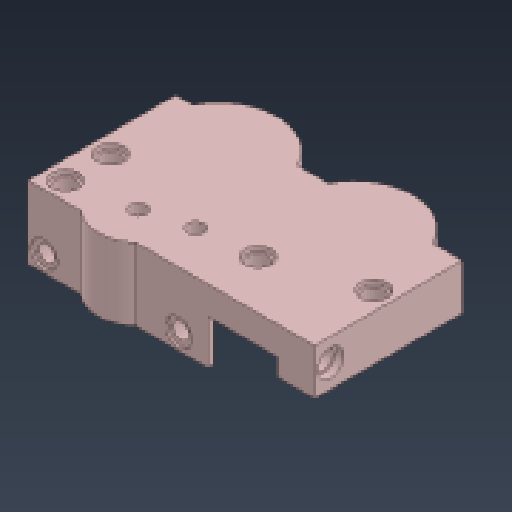
# Autodesk Inventor part: gearbox-holder-right
Saved by Autodesk Inventor 2023 (Build 270158000, 158)
## iProperties
Created: 2025-04-06
Part Number: gearbox-holder-right
Material: ABS Plastic
Document SubType Name: Modeling
Designer: szymo
Density: 1.06 g/cm^3
Appearance: Default(1)
Mass: 8.8839 g
Surface Area: 69.2878 cm^2
Volume: 8.38104 cm^3
Author: szymo
Autodesk Inventor part; units mm, degrees
(part 1 of 3)
ref_plane "YZ Plane" through (0, 0, 0) normal (1, 0, 0) x (0, 1, 0)
ref_plane "XZ Plane" through (0, 0, 0) normal (0, 1, 0) x (-1, 0, 0)
ref_plane "XY Plane" through (0, 0, 0) normal (0, 0, 1) x (1, 0, 0)
ref_plane "Work Plane1" through (-2.05, 16.2, 13.85) normal (0, 1, 0) x (0.7160287, 0, -0.6980708)
sketch "Sketch1" plane through (-2.05, 16.2, 13.85) normal (0, 1, 0) x (0.7160287, 0, -0.6980708)
  line L0 (-0.2487, 19.5853) -> (0.8969, 18.4684) projected
  line L1 (-18.9501, -1.8892) -> (0.8969, 18.4684) projected
  line L2 (-20.0957, -0.7723) -> (-18.9501, -1.8892) projected
  line L3 (-20.0957, -0.7723) -> (-0.2487, 19.5853) projected
  circle A0 centre (0, 8) radius 1.0564 projected
  circle A1 centre (0, -8) radius 1.0564 projected
  circle A2 centre (0, 0) radius 5 projected
  circle A3 centre (0, 0) radius 13.85 projected
  line L4 (0.8969, 18.4684) -> (19.5853, 0.2487)
  line L5 (19.5853, 0.2487) -> (0.2487, -19.5853)
  line L6 (0, 0) -> (9.917, -9.6683) construction
  circle A4 centre (19.834, -19.3366) radius 13.85 projected
  line L7 (19.5853, 0.2487) -> (25.0919, -5.1198)
  circle A5 centre (19.834, -19.3366) radius 14.25
  line L8 (25.0919, -5.1198) -> (24.3938, -5.8358)
  circle A6 centre (-3.741, -7.91) radius 1.25 projected
  arc A7 (-6.4074, -14.111) -> (-5.6342, -13.2068) centre (-9.5026, -10.6812) ccw projected
  arc A8 (-5.6342, -13.2068) -> (-5.2978, -13.3152) centre (-3.741, -7.91) ccw projected
  arc A9 (-5.2978, -13.3152) -> (-5.1983, -14.5008) centre (-0.6827, -13.5245) ccw projected
  arc A10 (-5.1983, -14.5008) -> (-4.7815, -14.5793) centre (-3.741, -7.91) ccw projected
  arc A11 (-4.7815, -14.5793) -> (-4.2574, -13.5112) centre (-8.6325, -12.027) ccw projected
  arc A12 (-4.2574, -13.5112) -> (-3.9047, -13.5326) centre (-3.741, -7.91) ccw projected
  arc A13 (-3.9047, -13.5326) -> (-3.5134, -14.6561) centre (0.6175, -12.5875) ccw projected
  arc A14 (-3.5134, -14.6561) -> (-3.0903, -14.6285) centre (-3.741, -7.91) ccw projected
  arc A15 (-3.0903, -14.6285) -> (-2.8482, -13.4637) centre (-7.4549, -13.1141) ccw projected
  arc A16 (-2.8482, -13.4637) -> (-2.5013, -13.3966) centre (-3.741, -7.91) ccw projected
  arc A17 (-2.5013, -13.3966) -> (-1.8429, -14.3876) centre (1.6439, -11.3566) ccw projected
  arc A18 (-1.8429, -14.3876) -> (-1.4399, -14.2556) centre (-3.741, -7.91) ccw projected
  arc A19 (-1.4399, -14.2556) -> (-1.4951, -13.0672) centre (-6.044, -13.8742) ccw projected
  arc A20 (-1.4951, -13.0672) -> (-1.1757, -12.916) centre (-3.741, -7.91) ccw projected
  arc A21 (-1.1757, -12.916) -> (-0.2916, -13.712) centre (2.3318, -9.9092) ccw projected
  arc A22 (-0.2916, -13.712) -> (0.0659, -13.484) centre (-3.741, -7.91) ccw projected
  arc A23 (0.0659, -13.484) -> (-0.2831, -12.3466) centre (-4.4884, -14.2596) ccw projected
  arc A24 (-0.2831, -12.3466) -> (-0.0114, -12.1207) centre (-3.741, -7.91) ccw projected
  arc A25 (-0.0114, -12.1207) -> (1.043, -12.6719) centre (2.6382, -8.3361) ccw projected
  arc A26 (1.043, -12.6719) -> (1.3325, -12.3621) centre (-3.741, -7.91) ccw projected
  arc A27 (1.3325, -12.3621) -> (0.7116, -11.3473) centre (-2.8859, -14.246) ccw projected
  arc A28 (0.7116, -11.3473) -> (0.9186, -11.0609) centre (-3.741, -7.91) ccw projected
  arc A29 (0.9186, -11.0609) -> (2.0769, -11.3326) centre (2.5438, -6.7363) ccw projected
  arc A30 (2.0769, -11.3326) -> (2.2804, -10.9605) centre (-3.741, -7.91) ccw projected
  arc A31 (2.2804, -10.9605) -> (1.4265, -10.132) centre (-1.337, -13.8342) ccw projected
  arc A32 (1.4265, -10.132) -> (1.5558, -9.8031) centre (-3.741, -7.91) ccw projected
  arc A33 (1.5558, -9.8031) -> (2.7453, -9.7782) centre (2.0545, -5.2102) ccw projected
  arc A34 (2.7453, -9.7782) -> (2.8498, -9.3672) centre (-3.741, -7.91) ccw projected
  arc A35 (2.8498, -9.3672) -> (1.8168, -8.7771) centre (0.0608, -13.0503) ccw projected
  arc A36 (1.8168, -8.7771) -> (1.8602, -8.4264) centre (-3.741, -7.91) ccw projected
  arc A37 (1.8602, -8.4264) -> (3.0061, -8.1064) centre (1.201, -3.8537) ccw projected
  arc A38 (3.0061, -8.1064) -> (3.0052, -7.6824) centre (-3.741, -7.91) ccw projected
  arc A39 (3.0052, -7.6824) -> (1.8578, -7.3677) centre (1.2197, -11.9433) ccw projected
  arc A40 (1.8578, -7.3677) -> (1.8127, -7.0172) centre (-3.741, -7.91) ccw projected
  arc A41 (1.8127, -7.0172) -> (2.843, -6.4223) centre (0.037, -2.7521) ccw projected
  arc A42 (2.843, -6.4223) -> (2.7366, -6.0118) centre (-3.741, -7.91) ccw projected
  arc A43 (2.7366, -6.0118) -> (1.547, -5.9923) centre (2.0669, -10.5829) ccw projected
  arc A44 (1.547, -5.9923) -> (1.4162, -5.6641) centre (-3.741, -7.91) ccw projected
  arc A45 (1.4162, -5.6641) -> (2.2662, -4.8317) centre (-1.3644, -1.9746) ccw projected
  arc A46 (2.2662, -4.8317) -> (2.0611, -4.4605) centre (-3.741, -7.91) ccw projected
  arc A47 (2.0611, -4.4605) -> (0.904, -4.7375) centre (2.5492, -9.0546) ccw projected
  arc A48 (0.904, -4.7375) -> (0.6957, -4.4521) centre (-3.741, -7.91) ccw projected
  arc A49 (0.6957, -4.4521) -> (1.3119, -3.4344) centre (-2.9151, -1.5701) ccw projected
  arc A50 (1.3119, -3.4344) -> (1.0209, -3.126) centre (-3.741, -7.91) ccw projected
  arc A51 (1.0209, -3.126) -> (-0.0309, -3.682) centre (2.6362, -7.4544) ccw projected
  arc A52 (-0.0309, -3.682) -> (-0.3037, -3.4574) centre (-3.741, -7.91) ccw projected
  arc A53 (-0.3037, -3.4574) -> (0.0402, -2.3184) centre (-4.5177, -1.5639) ccw projected
  arc A54 (0.0402, -2.3184) -> (-0.3184, -2.092) centre (-3.741, -7.91) ccw projected
  arc A55 (-0.3184, -2.092) -> (-1.1989, -2.8922) centre (2.3225, -5.8827) ccw projected
  arc A56 (-1.1989, -2.8922) -> (-1.519, -2.7424) centre (-3.741, -7.91) ccw projected
  arc A57 (-1.519, -2.7424) -> (-1.4692, -1.5538) centre (-6.0715, -1.9564) ccw projected
  arc A58 (-1.4692, -1.5538) -> (-1.8728, -1.4236) centre (-3.741, -7.91) ccw projected
  arc A59 (-1.8728, -1.4236) -> (-2.5266, -2.4176) centre (1.6279, -4.4385) ccw projected
  arc A60 (-2.5266, -2.4176) -> (-2.8739, -2.3522) centre (-3.741, -7.91) ccw projected
  arc A61 (-2.8739, -2.3522) -> (-3.1213, -1.1885) centre (-7.4789, -2.723) ccw projected
  arc A62 (-3.1213, -1.1885) -> (-3.5445, -1.1628) centre (-3.741, -7.91) ccw projected
  arc A63 (-3.5445, -1.1628) -> (-3.9307, -2.2882) centre (0.5959, -3.2123) ccw projected
  arc A64 (-3.9307, -2.2882) -> (-4.2833, -2.3112) centre (-3.741, -7.91) ccw projected
  arc A65 (-4.2833, -2.3112) -> (-4.8123, -1.2455) centre (-8.6514, -3.8156) ccw projected
  arc A66 (-4.8123, -1.2455) -> (-5.2287, -1.3259) centre (-3.741, -7.91) ccw projected
  arc A67 (-5.2287, -1.3259) -> (-5.3228, -2.5119) centre (-0.7086, -2.2814) ccw projected
  arc A68 (-5.3228, -2.5119) -> (-5.6586, -2.6219) centre (-3.741, -7.91) ccw projected
  arc A69 (-5.6586, -2.6219) -> (-6.436, -1.7213) centre (-9.5154, -5.1654) ccw projected
  arc A70 (-6.436, -1.7213) -> (-6.8193, -1.9028) centre (-3.741, -7.91) ccw projected
  arc A71 (-6.8193, -1.9028) -> (-6.6155, -3.0749) centre (-2.2036, -1.7041) ccw projected
  arc A72 (-6.6155, -3.0749) -> (-6.9134, -3.2649) centre (-3.741, -7.91) ccw projected
  arc A73 (-6.9134, -3.2649) -> (-7.8904, -2.586) centre (-10.0165, -6.6876) ccw projected
  arc A74 (-7.8904, -2.586) -> (-8.2165, -2.857) centre (-3.741, -7.91) ccw projected
  arc A75 (-8.2165, -2.857) -> (-7.7276, -3.9417) centre (-3.7953, -1.5167) ccw projected
  arc A76 (-7.7276, -3.9417) -> (-7.9689, -4.1998) centre (-3.741, -7.91) ccw projected
  arc A77 (-7.9689, -4.1998) -> (-9.0841, -3.7852) centre (-10.1233, -8.2867) ccw projected
  arc A78 (-9.0841, -3.7852) -> (-9.3325, -4.1288) centre (-3.741, -7.91) ccw projected
  arc A79 (-9.3325, -4.1288) -> (-8.5893, -5.0578) centre (-5.3835, -1.7311) ccw projected
  arc A80 (-8.5893, -5.0578) -> (-8.7588, -5.3678) centre (-3.741, -7.91) ccw projected
  arc A81 (-8.7588, -5.3678) -> (-9.942, -5.2435) centre (-9.8291, -9.8621) ccw projected
  arc A82 (-9.942, -5.2435) -> (-10.0972, -5.6381) centre (-3.741, -7.91) ccw projected
  arc A83 (-10.0972, -5.6381) -> (-9.1463, -6.3531) centre (-6.8685, -2.3337) ccw projected
  arc A84 (-9.1463, -6.3531) -> (-9.2333, -6.6956) centre (-3.741, -7.91) ccw projected
  arc A85 (-9.2333, -6.6956) -> (-10.4103, -6.8694) centre (-9.1524, -11.3148) ccw projected
  arc A86 (-10.4103, -6.8694) -> (-10.4625, -7.2902) centre (-3.741, -7.91) ccw projected
  arc A87 (-10.4625, -7.2902) -> (-9.3636, -7.7462) centre (-8.157, -3.2867) ccw projected
  arc A88 (-9.3636, -7.7462) -> (-9.3628, -8.0996) centre (-3.741, -7.91) ccw projected
  arc A89 (-9.3628, -8.0996) -> (-10.4596, -8.5607) centre (-8.1356, -12.5536) ccw projected
  arc A90 (-10.4596, -8.5607) -> (-10.4054, -8.9813) centre (-3.741, -7.91) ccw projected
  arc A91 (-10.4054, -8.9813) -> (-9.2277, -9.1497) centre (-9.1681, -4.5301) ccw projected
  arc A92 (-9.2277, -9.1497) -> (-9.139, -9.4917) centre (-3.741, -7.91) ccw projected
  arc A93 (-9.139, -9.4917) -> (-10.0866, -10.2111) centre (-6.8427, -13.5006) ccw projected
  arc A94 (-10.0866, -10.2111) -> (-9.9296, -10.605) centre (-3.741, -7.91) ccw projected
  arc A95 (-9.9296, -10.605) -> (-8.747, -10.4752) centre (-9.8381, -5.986) ccw projected
  arc A96 (-8.747, -10.4752) -> (-8.576, -10.7845) centre (-3.741, -7.91) ccw projected
  arc A97 (-8.576, -10.7845) -> (-9.315, -11.7169) centre (-5.355, -14.0963) ccw projected
  arc A98 (-9.315, -11.7169) -> (-9.065, -12.0594) centre (-3.741, -7.91) ccw projected
  arc A99 (-9.065, -12.0594) -> (-7.9518, -11.6396) centre (-10.125, -7.5627) ccw projected
  arc A100 (-7.9518, -11.6396) -> (-7.7093, -11.8966) centre (-3.741, -7.91) ccw projected
  arc A101 (-7.7093, -11.8966) -> (-8.1932, -12.9835) centre (-3.7658, -14.3034) ccw projected
  arc A102 (-8.1932, -12.9835) -> (-7.8658, -13.253) centre (-3.741, -7.91) ccw projected
  arc A103 (-7.8658, -13.253) -> (-6.892, -12.5696) centre (-10.0108, -9.1613) ccw projected
  arc A104 (-6.892, -12.5696) -> (-6.5932, -12.7582) centre (-3.741, -7.91) ccw projected
  arc A105 (-6.5932, -12.7582) -> (-6.7915, -13.9313) centre (-2.175, -14.1087) ccw projected
  arc A106 (-6.7915, -13.9313) -> (-6.4074, -14.111) centre (-3.741, -7.91) ccw projected
  circle A107 centre (-3.741, -7.91) radius 6.75
  circle A108 centre (-3.741, -7.91) radius 7.15
  circle A109 centre (-3.741, -7.91) radius 7.55
  line L9 (-18.4396, -1.3656) -> (10.1657, -29.2536)
  line L10 (19.834, -19.3366) -> (10.1657, -29.2536)
  line L11 (6.4534, -24.2377) -> (5.7553, -24.9538)
  circle A110 centre (0, -8) radius 1.4564
  circle A111 centre (0, 8) radius 1.4564
  circle A112 centre (0, 0) radius 5.4
  point P0 (11.1361, 8.486)
  point P1 (-8.0316, -13.1208)
  point P2 (-5.3731, -0.5385)
  point P3 (2.9925, -4.495)
  point P4 (-11.2783, -8.3473)
  point P5 (-3.9868, -15.456)
  point P6 (2.2948, -4.8881)
  point P7 (2.2662, -4.8317)
  point P8 (2.1767, -4.9419)
  point P9 (-5.2314, -1.3389)
  point P10 (-5.2287, -1.3259)
  point P11 (-5.2344, -1.3272)
  point P12 (7.5766, -12.0688)
  point P13 (12.2574, -7.2677)
  point P14 (7.7651, -26.9132)
  dimension "d0" = 0
  dimension "d3" = 0.4
  dimension "d5" = 1
  dimension "d6" = 0.4
  dimension "d7" = 0.4
  dimension "d9" = 1
  dimension "d10" = 0.4
  dimension "d11" = 0.4
  dimension "d12" = 0.4
  constraints: 16 end point, 6 centre point, 4 perpendicular, 3 parallel, 3 point on circle, 3 point on line, 1 coincident, 1 collinear, 7 other
  measures "d0" distance from line of L6.end L5
  measures "d5" distance of L7.end L8.end
  measures "d7" radial gap between concentric circles of A108 A109
  measures "d9" distance of L11.start L11.end
  measures "d10" radial gap between concentric circles of A1 A110
  measures "d11" radial gap between concentric circles of A0 A111
  measures "d12" radial gap between concentric circles of A2 A112
extrude "Extrusion1" add sketch "Sketch1" along normal blind 3.1 contours L4 A3 L1 | A3 A5 A109 A112 L1 | L4 L5 A5 A3 | A3 A109 L9 L1 | L7 L8 A5 L5 | A109 A112 A108 A3 | A3 A108 L9 A109 | L9 A108 A109 | A108 A112 A107 A70 A74 A78 A82 A86 A90 A3 | A3 A107 L9 A108 | A5 L5 L9 A109 A3 | L9 A108 A3 A109 | L9 A107 A94 A98 A102 A106 A10 A108 | A107 A91 A92 A93 A3 | A3 L9 A107 | A5 L11 L9 L5 | A3 A108 A112 A109 | L9 A10 A107 A14 A18 A3 A108 | L9 A93 A107 | A93 A92 A91 A90 A89 A88 A87 A86 A85 A84 A83 A82 A81 A80 A79 A78 A77 A76 A75 A74 A73 A72 A71 A70 A69 A68 A67 A112 A45 A44 A43 A42 A41 A40 A39 A38 A37 A36 A35 A34 A33 A32 A31 A30 A29 A28 A27 A26 A25 A24 A23 A22 A21 A20 A19 A3 A17 A16 A15 A97 A96 A95 | L9 A95 A94 A93 | A3 A95 L9 | A112 A67 A68 A69 A107 | A107 A67 A112 | A3 A107 A22 A26 A30 A34 A38 A42 A112 A108 | L9 A9 A8 A7 A105 A104 A103 A97 A3 A15 A14 A13 A12 A11 A10 | A10 A9 L9 | A95 A96 A97 A3 | A3 A97 L9 A95 | L9 A97 A107 A95 | A107 A87 A88 A89 | A107 A19 A3 | A3 A19 A20 A21 A107 | A107 A7 L9 A9 | A11 A12 A13 A107 | L9 A7 A8 A9 | L9 A103 A102 A101 A100 A99 A98 A97 | A71 A72 A73 A107 | A112 A107 A43 A44 A45 | A19 A18 A17 A3 | A106 A105 L9 A7 | A15 A16 A17 A3 | A3 A17 A107 A15 | L9 A105 A107 A103 | A103 A104 A105 L9 | A107 A83 A84 A85 | A23 A24 A25 A107 | A99 A100 A101 A107 | A75 A76 A77 A107 | A107 A39 A40 A41 | A107 A79 A80 A81 | A27 A28 A29 A107 | A107 A35 A36 A37 | A31 A32 A33 A107 | A0 | A1 | A6 | A110 | A111
ref_plane "Work Plane7" through (-20.9, 49.5, 14.2156) normal (0, 1, 0) x (-1, 0, 0)
ref_plane "Work Plane2" through (-20.9, 49.5, 14.2156) normal (0, 1, 0) x (-1, 0, 0)
ref_plane "Work Plane3" through (-4.2986, 19.3, 27.7) normal (0, 1, 0) x (-1, 0, 0)
sketch "Sketch2" plane through (-4.2986, 19.3, 27.7) normal (0, 1, 0) x (-1, 0, 0)
  circle A0 centre (-2.9986, -22.8337) radius 4 projected
  circle A1 centre (-2.9986, -22.8337) radius 4.2
  point P0 (-4.2986, -27.7)
  dimension "d15" = 0.2
  constraints: 1 centre point
  measures "d15" radial gap between concentric circles of A0 A1
extrude "Extrusion2" cut sketch "Sketch2" against normal blind 0.6 contours A0 | A1
sketch "Sketch3" plane through (-4.2986, 19.3, 27.7) normal (0, 1, 0) x (-1, 0, 0)
  arc A0 (0.5626, -9.2394) -> (-4.3064, -18.8425) centre (-2.2486, -13.85) ccw projected
  arc A1 (0.5697, -9.2506) -> (0.5626, -9.2394) centre (-3.3337, -11.7218) ccw projected
  arc A2 (0.5697, -9.2506) -> (0.5729, -9.2457) centre (-5.0916, -5.5748) ccw projected
  line L0 (-23.789, -27.7) -> (10.0014, -27.7) projected
  line L1 (10.0014, -27.7) -> (10.0014, 0) projected
  line L2 (10.0014, 0) -> (0, 0) projected
  arc A3 (0, 0) -> (-10.1832, 0) centre (-5.0916, -5.5748) ccw projected
  line L3 (-10.1832, 0) -> (-23.789, 0) projected
  arc A4 (-23.789, -26.7) -> (-23.789, -1) centre (-29.9486, -13.85) ccw projected
  line L4 (-23.789, -26.7) -> (-23.789, -27.7) projected
  circle A5 centre (-5.0916, -5.5748) radius 7.15
  arc A6 (-4.3064, -18.8425) -> (-1.0471, -19.1146) centre (-2.9986, -22.8337) ccw projected
  arc A7 (-1.0471, -19.1146) -> (0.5729, -9.2457) centre (-2.2486, -13.85) ccw projected
  line L5 (-23.789, 0) -> (-23.789, -1) projected
  point P0 (-4.2986, -27.7)
  point P1 (-7.4306, -12.3314)
  point P2 (0.906, -9.4672)
  point P3 (0.906, -9.4672)
  dimension "d18" = 0.4
  constraints: 1 centre point, 1 coincident
  measures "d18" radial gap between concentric circles of A3 A5
extrude "Extrusion3" add sketch "Sketch3" along normal blind 2.6
ref_plane "Work Plane4" through (30.4216, 21.2, 8.0637) normal (0, 1, 0) x (-1, 0, 0)
sketch "Sketch5" plane through (30.4216, 21.2, 8.0637) normal (0, 1, 0) x (-1, 0, 0)
  line L0 (10.9312, -8.0637) -> (44.7216, -8.0637) projected
  line L1 (44.7216, -8.0637) -> (44.7216, 19.6363) projected
  line L2 (44.7216, 19.6363) -> (34.7202, 19.6363) projected
  arc A0 (34.7202, 19.6363) -> (24.537, 19.6363) centre (29.6286, 14.0616) ccw projected
  line L3 (24.537, 19.6363) -> (10.9312, 19.6363) projected
  arc A1 (10.9312, -7.0637) -> (10.9312, 18.6363) centre (4.7716, 5.7863) ccw projected
  line L4 (10.9312, -7.0637) -> (10.9312, -8.0637) projected
  circle A2 centre (21.2038, 11.6981) radius 1.25 projected
  arc A3 (24.6098, 5.8704) -> (24.3415, 7.0295) centre (20.0122, 5.4167) ccw projected
  arc A4 (24.3415, 7.0295) -> (24.6284, 7.2357) centre (21.2038, 11.6981) ccw projected
  arc A5 (24.6284, 7.2357) -> (25.6415, 6.6119) centre (27.5374, 10.8249) ccw projected
  arc A6 (25.6415, 6.6119) -> (25.9521, 6.9006) centre (21.2038, 11.6981) ccw projected
  arc A7 (25.9521, 6.9006) -> (25.4039, 7.9565) centre (21.6118, 5.3177) ccw projected
  arc A8 (25.4039, 7.9565) -> (25.6306, 8.2276) centre (21.2038, 11.6981) ccw projected
  arc A9 (25.6306, 8.2276) -> (26.767, 7.8753) centre (27.5555, 12.4274) ccw projected
  arc A10 (26.767, 7.8753) -> (26.996, 8.2321) centre (21.2038, 11.6981) ccw projected
  arc A11 (26.996, 8.2321) -> (26.2025, 9.1186) centre (23.1857, 5.6196) ccw projected
  arc A12 (26.2025, 9.1186) -> (26.3546, 9.4375) centre (21.2038, 11.6981) ccw projected
  arc A13 (26.3546, 9.4375) -> (27.5429, 9.3789) centre (27.1746, 13.9841) ccw projected
  arc A14 (27.5429, 9.3789) -> (27.676, 9.7815) centre (21.2038, 11.6981) ccw projected
  arc A15 (27.676, 9.7815) -> (26.6869, 10.4427) centre (24.6351, 6.3034) ccw projected
  arc A16 (26.6869, 10.4427) -> (26.7549, 10.7895) centre (21.2038, 11.6981) ccw projected
  arc A17 (26.7549, 10.7895) -> (27.9205, 11.0282) centre (26.4185, 15.3972) ccw projected
  arc A18 (27.9205, 11.0282) -> (27.9493, 11.4513) centre (21.2038, 11.6981) ccw projected
  arc A19 (27.9493, 11.4513) -> (26.8269, 11.8458) centre (25.8689, 7.3262) ccw projected
  arc A20 (26.8269, 11.8458) -> (26.8065, 12.1986) centre (21.2038, 11.6981) ccw projected
  arc A21 (26.8065, 12.1986) -> (27.8761, 12.7196) centre (25.3348, 16.5778) ccw projected
  arc A22 (27.8761, 12.7196) -> (27.7988, 13.1365) centre (21.2038, 11.6981) ccw projected
  arc A23 (27.7988, 13.1365) -> (26.6135, 13.2395) centre (26.8096, 8.6238) ccw projected
  arc A24 (26.6135, 13.2395) -> (26.506, 13.5762) centre (21.2038, 11.6981) ccw projected
  arc A25 (26.506, 13.5762) -> (27.4124, 14.3468) centre (23.9915, 17.4518) ccw projected
  arc A26 (27.4124, 14.3468) -> (27.2338, 14.7315) centre (21.2038, 11.6981) ccw projected
  arc A27 (27.2338, 14.7315) -> (26.0602, 14.5364) centre (27.398, 10.1144) ccw projected
  arc A28 (26.0602, 14.5364) -> (25.8724, 14.8358) centre (21.2038, 11.6981) ccw projected
  arc A29 (25.8724, 14.8358) -> (26.5586, 15.8076) centre (22.473, 17.9643) ccw projected
  arc A30 (26.5586, 15.8076) -> (26.29, 16.1358) centre (21.2038, 11.6981) ccw projected
  arc A31 (26.29, 16.1358) -> (25.2018, 15.655) centre (27.5973, 11.7046) ccw projected
  arc A32 (25.2018, 15.655) -> (24.9454, 15.8982) centre (21.2038, 11.6981) ccw projected
  arc A33 (24.9454, 15.8982) -> (25.3684, 17.0102) centre (20.8748, 18.0831) ccw projected
  arc A34 (25.3684, 17.0102) -> (25.0266, 17.2612) centre (21.2038, 11.6981) ccw projected
  arc A35 (25.0266, 17.2612) -> (24.0921, 16.5249) centre (27.3948, 13.2944) ccw projected
  arc A36 (24.0921, 16.5249) -> (23.7833, 16.6968) centre (21.2038, 11.6981) ccw projected
  arc A37 (23.7833, 16.6968) -> (23.9165, 17.879) centre (19.2972, 17.8006) ccw projected
  arc A38 (23.9165, 17.879) -> (23.523, 18.0372) centre (21.2038, 11.6981) ccw projected
  arc A39 (23.523, 18.0372) -> (22.801, 17.0916) centre (26.8033, 14.7839) ccw projected
  arc A40 (22.801, 17.0916) -> (22.4592, 17.1812) centre (21.2038, 11.6981) ccw projected
  arc A41 (22.4592, 17.1812) -> (22.2941, 18.3595) centre (17.8395, 17.1348) ccw projected
  arc A42 (22.2941, 18.3595) -> (21.8737, 18.4148) centre (21.2038, 11.6981) ccw projected
  arc A43 (21.8737, 18.4148) -> (21.4095, 17.3193) centre (25.86, 16.0795) ccw projected
  arc A44 (21.4095, 17.3193) -> (21.0561, 17.3212) centre (21.2038, 11.6981) ccw projected
  arc A45 (21.0561, 17.3212) -> (20.6033, 18.4213) centre (16.5931, 16.1273) ccw projected
  arc A46 (20.6033, 18.4213) -> (20.1823, 18.3704) centre (21.2038, 11.6981) ccw projected
  arc A47 (20.1823, 18.3704) -> (20.0051, 17.1939) centre (24.6241, 17.0998) ccw projected
  arc A48 (20.0051, 17.1939) -> (19.6624, 17.1078) centre (21.2038, 11.6981) ccw projected
  arc A49 (19.6624, 17.1078) -> (18.9501, 18.0608) centre (15.6365, 14.8415) ccw projected
  arc A50 (18.9501, 18.0608) -> (18.5551, 17.9067) centre (21.2038, 11.6981) ccw projected
  arc A51 (18.5551, 17.9067) -> (18.676, 16.7231) centre (23.1733, 17.7806) ccw projected
  arc A52 (18.676, 16.7231) -> (18.3655, 16.5545) centre (21.2038, 11.6981) ccw projected
  arc A53 (18.3655, 16.5545) -> (17.4386, 17.3004) centre (15.0297, 13.3582) ccw projected
  arc A54 (17.4386, 17.3004) -> (17.0943, 17.0529) centre (21.2038, 11.6981) ccw projected
  arc A55 (17.0943, 17.0529) -> (17.5058, 15.9366) centre (21.5987, 18.0793) ccw projected
  arc A56 (17.5058, 15.9366) -> (17.2469, 15.696) centre (21.2038, 11.6981) ccw projected
  arc A57 (17.2469, 15.696) -> (16.1637, 16.188) centre (14.8108, 11.7706) ccw projected
  arc A58 (16.1637, 16.188) -> (15.8917, 15.8627) centre (21.2038, 11.6981) ccw projected
  arc A59 (15.8917, 15.8627) -> (16.5679, 14.8838) centre (19.9994, 17.9771) ccw projected
  arc A60 (16.5679, 14.8838) -> (16.377, 14.5864) centre (21.2038, 11.6981) ccw projected
  arc A61 (16.377, 14.5864) -> (15.2054, 14.7935) centre (14.9936, 10.1785) ccw projected
  arc A62 (15.2054, 14.7935) -> (15.0229, 14.4108) centre (21.2038, 11.6981) ccw projected
  arc A63 (15.0229, 14.4108) -> (15.9213, 13.6308) centre (18.4757, 17.4803) ccw projected
  arc A64 (15.9213, 13.6308) -> (15.8103, 13.2953) centre (21.2038, 11.6981) ccw projected
  arc A65 (15.8103, 13.2953) -> (14.6241, 13.2045) centre (15.5666, 8.6818) ccw projected
  arc A66 (14.6241, 13.2045) -> (14.5425, 12.7884) centre (21.2038, 11.6981) ccw projected
  arc A67 (14.5425, 12.7884) -> (15.6066, 12.2563) centre (17.1234, 16.6202) ccw projected
  arc A68 (15.6066, 12.2563) -> (15.5826, 11.9038) centre (21.2038, 11.6981) ccw projected
  arc A69 (15.5826, 11.9038) -> (14.4561, 11.5209) centre (16.4938, 7.3746) ccw projected
  arc A70 (14.4561, 11.5209) -> (14.4806, 11.0976) centre (21.2038, 11.6981) ccw projected
  arc A71 (14.4806, 11.0976) -> (15.6436, 10.8468) centre (16.0276, 15.4508) ccw projected
  arc A72 (15.6436, 10.8468) -> (15.708, 10.4994) centre (21.2038, 11.6981) ccw projected
  arc A73 (15.708, 10.4994) -> (14.7122, 9.8484) centre (17.717, 6.3391) ccw projected
  arc A74 (14.7122, 9.8484) -> (14.8412, 9.4444) centre (21.2038, 11.6981) ccw projected
  arc A75 (14.8412, 9.4444) -> (16.03, 9.4908) centre (15.2569, 14.0456) ccw projected
  arc A76 (16.03, 9.4908) -> (16.1788, 9.1703) centre (21.2038, 11.6981) ccw projected
  arc A77 (16.1788, 9.1703) -> (15.3761, 8.2921) centre (19.1593, 5.6404) ccw projected
  arc A78 (15.3761, 8.2921) -> (15.6015, 7.9329) centre (21.2038, 11.6981) ccw projected
  arc A79 (15.6015, 7.9329) -> (16.7415, 8.2735) centre (14.86, 12.4929) ccw projected
  arc A80 (16.7415, 8.2735) -> (16.9653, 8) centre (21.2038, 11.6981) ccw projected
  arc A81 (16.9653, 8) -> (16.4063, 6.9498) centre (20.73, 5.3222) ccw projected
  arc A82 (16.4063, 6.9498) -> (16.7139, 6.6579) centre (21.2038, 11.6981) ccw projected
  arc A83 (16.7139, 6.6579) -> (17.7333, 7.2713) centre (14.8616, 10.8903) ccw projected
  arc A84 (17.7333, 7.2713) -> (18.0181, 7.0621) centre (21.2038, 11.6981) ccw projected
  arc A85 (18.0181, 7.0621) -> (17.7378, 5.9059) centre (22.3305, 5.4047) ccw projected
  arc A86 (17.7378, 5.9059) -> (18.1084, 5.6997) centre (21.2038, 11.6981) ccw projected
  arc A87 (18.1084, 5.6997) -> (18.9432, 6.5473) centre (15.2617, 9.3384) ccw projected
  arc A88 (18.9432, 6.5473) -> (19.2711, 6.4155) centre (21.2038, 11.6981) ccw projected
  arc A89 (19.2711, 6.4155) -> (19.2872, 5.2259) centre (23.8602, 5.8826) ccw projected
  arc A90 (19.2872, 5.2259) -> (19.6974, 5.1183) centre (21.2038, 11.6981) ccw projected
  arc A91 (19.6974, 5.1183) -> (20.2952, 6.147) centre (16.0352, 7.9348) ccw projected
  arc A92 (20.2952, 6.147) -> (20.6456, 6.1009) centre (21.2038, 11.6981) ccw projected
  arc A93 (20.6456, 6.1009) -> (20.957, 4.9526) centre (25.223, 6.7259) ccw projected
  arc A94 (20.957, 4.9526) -> (21.381, 4.9504) centre (21.2038, 11.6981) ccw projected
  arc A95 (21.381, 4.9504) -> (21.7043, 6.0954) centre (17.1335, 6.7677) ccw projected
  arc A96 (21.7043, 6.0954) -> (22.0551, 6.1379) centre (21.2038, 11.6981) ccw projected
  arc A97 (22.0551, 6.1379) -> (22.6423, 5.1031) centre (26.3333, 7.8817) ccw projected
  arc A98 (22.6423, 5.1031) -> (23.0535, 5.2065) centre (21.2038, 11.6981) ccw projected
  arc A99 (23.0535, 5.2065) -> (23.0819, 6.3959) centre (18.4875, 5.9103) ccw projected
  arc A100 (23.0819, 6.3959) -> (23.4111, 6.5243) centre (21.2038, 11.6981) ccw projected
  arc A101 (23.4111, 6.5243) -> (24.2372, 5.6681) centre (27.1212, 9.2772) ccw projected
  arc A102 (24.2372, 5.6681) -> (24.6098, 5.8704) centre (21.2038, 11.6981) ccw projected
  circle A103 centre (21.2038, 11.6981) radius 6.75
  circle A104 centre (21.2038, 11.6981) radius 7.15
  circle A105 centre (21.2038, 11.6981) radius 7.75
  line L5 (1.2537, -0.8374) -> (-1.3251, -3.9646) projected
  arc A106 (-3.6396, -2.0559) -> (-1.3251, -3.9646) centre (4.7716, 5.7863) ccw projected
  line L6 (-3.6396, -2.0559) -> (-1.0609, 1.0712) projected
  arc A107 (-1.0609, 1.0712) -> (1.2537, -0.8374) centre (4.7716, 5.7863) ccw projected
  arc A108 (13.1829, 13.6286) -> (10.8683, 15.5372) centre (4.7716, 5.7863) ccw projected
  line L7 (13.1829, 13.6286) -> (10.6041, 10.5014) projected
  arc A109 (10.6041, 10.5014) -> (8.2896, 12.4101) centre (4.7716, 5.7863) ccw projected
  line L8 (8.2896, 12.4101) -> (10.8683, 15.5372) projected
  circle A110 centre (4.7716, 5.7863) radius 5 projected
  circle A111 centre (4.7716, 5.7863) radius 13.85 projected
  circle A112 centre (4.7716, 5.7863) radius 5.4
  line L9 (-9.0784, 22.3676) -> (-9.0784, -10.0637) projected
  line L10 (-9.0784, 22.3676) -> (-11.0784, 22.3676) projected
  line L11 (-11.0784, -8.0637) -> (-11.0784, 22.3676) projected
  line L12 (10.9312, -8.0637) -> (44.7216, -8.0637) projected
  line L13 (10.9312, -8.0637) -> (-9.0784, -8.0637)
  line L14 (8.1242, 19.6363) -> (-9.0784, 19.6363)
  line L15 (-9.0784, 19.6363) -> (-9.0784, -8.0637)
  arc A113 (14.2335, 13.6452) -> (10.6846, 16.5718) centre (4.7716, 5.7863) ccw
  line L16 (14.2335, 13.6452) -> (10.5497, 9.178)
  arc A114 (10.5497, 9.178) -> (7.0008, 12.1046) centre (4.7716, 5.7863) ccw
  line L17 (7.0008, 12.1046) -> (10.6846, 16.5718)
  line L18 (-1.0065, 2.3946) -> (-4.6903, -2.0726)
  arc A115 (-4.6903, -2.0726) -> (-1.1413, -4.9992) centre (4.7716, 5.7863) ccw
  line L19 (-1.1413, -4.9992) -> (2.5425, -0.532)
  arc A116 (-1.0065, 2.3946) -> (2.5425, -0.532) centre (4.7716, 5.7863) ccw
  line L20 (-4.6903, -2.0726) -> (-4.6903, 19.6363)
  line L21 (2.5425, -0.532) -> (2.5425, 0.8679)
  line L22 (2.5425, 0.8679) -> (2.5425, 19.6363)
  line L23 (7.0008, 12.1046) -> (7.0008, 19.6363)
  line L24 (13.8357, 14.1009) -> (13.8357, 19.6363)
  line L25 (10.5497, 9.178) -> (10.1716, 5.7863)
  line L26 (2.5425, -0.532) -> (3.2095, 0.6172)
  line L27 (10.9312, 19.6363) -> (10.9312, 18.6363) projected
  line L28 (-11.0784, -8.0637) -> (-9.0784, -10.0637) projected
  point P0 (30.4216, -8.0637)
  point P1 (14.7382, 15.9711)
  point P2 (18.9423, 4.2854)
  point P3 (13.8357, 16.2584)
  point P4 (14.5213, 15.6233)
  point P5 (13.5317, 12.7942)
  point P6 (13.8357, 16.782)
  point P7 (-9.0784, -8.0637)
  dimension "d25" = 0.4
  dimension "d26" = 0.6
  dimension "d29" = 0.4
  dimension "d30" = 0.8
  dimension "d31" = 0.8
  constraints: 28 end point, 12 point on circle, 6 centre point, 6 point on line, 4 perpendicular, 2 collinear, 1 coincident, 1 parallel, 12 other
  measures "d29" radial gap between concentric circles of A110 A112
  measures "d30" distance between parallel lines of L8 L17
  measures "d31" distance between parallel lines of L6 L18
extrude "Extrusion5" add sketch "Sketch5" along normal up to surface (0.7 mm away) contours L13 A111 A105 A1 L4 | L13 L9 A111 | A111 L20 A115 L19 L26 A112 L25 L16 A105 | A105 A111 A104 A1 | A1 A104 A105 | L9 L14 L20 A111 | A105 L16 A113 A111 A104 | A104 A111 A103 A1 | A1 A103 A90 A94 A98 A102 A6 A10 A14 A18 A22 A26 A30 A34 A38 A42 A46 A50 A54 A58 A104 | L16 A114 L17 A113 A105 | A105 A113 L16 | A104 A111 A103 A62 A66 A70 A74 A78 A82 A86 | A103 A111 A87 A88 A1 | A1 A88 A89 A103 | A105 A111 L24 A1 | A1 A104 A111 A105 | L24 A111 A105 | A104 A1 A103 A111 | A103 A87 A111 | A88 A87 A111 A61 A1 | A1 A61 A60 A59 A58 A57 A56 A55 A54 A53 A52 A51 A50 A49 A48 A47 A46 A45 A44 A43 A42 A41 A40 A39 A38 A37 A36 A35 A34 A33 A32 A31 A30 A29 A28 A27 A26 A25 A24 A23 A22 A21 A20 A19 A18 A17 A16 A15 A14 A13 A12 A11 A10 A9 A8 A7 A6 A5 A4 A3 A102 A101 A100 A99 A98 A97 A96 A95 A94 A93 A92 A91 A90 A89 A88 | A111 A61 A103 | A103 A1 A61 A111 | A86 A85 A84 A83 A82 A81 A80 A79 A78 A77 A76 A75 A74 A73 A72 A71 A70 A69 A68 A67 A66 A65 A64 A63 A62 A61 A111 A87 | A1 A103 A59 A60 A61 | A91 A92 A93 A103 | A103 A83 A84 A85 | A63 A64 A65 A103 | A95 A96 A97 A103 | A103 A55 A56 A57 | A103 A79 A80 A81 | A67 A68 A69 A103 | A99 A100 A101 A103 | A103 A51 A52 A53 | A103 A75 A76 A77 | A71 A72 A73 A103 | A3 A4 A5 A103 | A103 A47 A48 A49 | A7 A8 A9 A103 | A103 A43 A44 A45 | A11 A12 A13 A103 | A103 A39 A40 A41 | A15 A16 A17 A103 | A103 A35 A36 A37 | A19 A20 A21 A103 | A103 A31 A32 A33 | A103 A27 A28 A29 | A23 A24 A25 A103 | A2 | L7 A109 L8 A108
sketch "Sketch6" plane through (-4.2986, 21.9, 27.7) normal (0, 1, 0) x (1, 0, 0)
  circle A0 centre (13.5164, 7.9382) radius 1.25 projected
  arc A1 (10.1104, 13.7659) -> (10.3787, 12.6068) centre (14.708, 14.2197) ccw projected
  arc A2 (10.3787, 12.6068) -> (10.0917, 12.4006) centre (13.5164, 7.9382) ccw projected
  arc A3 (10.0917, 12.4006) -> (9.0787, 13.0245) centre (7.1828, 8.8114) ccw projected
  arc A4 (9.0787, 13.0245) -> (8.7681, 12.7358) centre (13.5164, 7.9382) ccw projected
  arc A5 (8.7681, 12.7358) -> (9.3162, 11.6798) centre (13.1084, 14.3187) ccw projected
  arc A6 (9.3162, 11.6798) -> (9.0896, 11.4087) centre (13.5164, 7.9382) ccw projected
  arc A7 (9.0896, 11.4087) -> (7.9532, 11.7611) centre (7.1646, 7.2089) ccw projected
  arc A8 (7.9532, 11.7611) -> (7.7242, 11.4042) centre (13.5164, 7.9382) ccw projected
  arc A9 (7.7242, 11.4042) -> (8.5177, 10.5178) centre (11.5345, 14.0167) ccw projected
  arc A10 (8.5177, 10.5178) -> (8.3656, 10.1988) centre (13.5164, 7.9382) ccw projected
  arc A11 (8.3656, 10.1988) -> (7.1773, 10.2575) centre (7.5456, 5.6522) ccw projected
  arc A12 (7.1773, 10.2575) -> (7.0442, 9.8549) centre (13.5164, 7.9382) ccw projected
  arc A13 (7.0442, 9.8549) -> (8.0332, 9.1936) centre (10.0851, 13.3329) ccw projected
  arc A14 (8.0332, 9.1936) -> (7.9652, 8.8468) centre (13.5164, 7.9382) ccw projected
  arc A15 (7.9652, 8.8468) -> (6.7997, 8.6081) centre (8.3017, 4.2392) ccw projected
  arc A16 (6.7997, 8.6081) -> (6.7709, 8.1851) centre (13.5164, 7.9382) ccw projected
  arc A17 (6.7709, 8.1851) -> (7.8933, 7.7906) centre (8.8513, 12.3101) ccw projected
  arc A18 (7.8933, 7.7906) -> (7.9137, 7.4378) centre (13.5164, 7.9382) ccw projected
  arc A19 (7.9137, 7.4378) -> (6.8441, 6.9167) centre (9.3854, 3.0585) ccw projected
  arc A20 (6.8441, 6.9167) -> (6.9214, 6.4998) centre (13.5164, 7.9382) ccw projected
  arc A21 (6.9214, 6.4998) -> (8.1067, 6.3968) centre (7.9106, 11.0126) ccw projected
  arc A22 (8.1067, 6.3968) -> (8.2142, 6.0602) centre (13.5164, 7.9382) ccw projected
  arc A23 (8.2142, 6.0602) -> (7.3078, 5.2895) centre (10.7287, 2.1845) ccw projected
  arc A24 (7.3078, 5.2895) -> (7.4863, 4.9049) centre (13.5164, 7.9382) ccw projected
  arc A25 (7.4863, 4.9049) -> (8.66, 5.0999) centre (7.3222, 9.5219) ccw projected
  arc A26 (8.66, 5.0999) -> (8.8478, 4.8006) centre (13.5164, 7.9382) ccw projected
  arc A27 (8.8478, 4.8006) -> (8.1615, 3.8287) centre (12.2472, 1.672) ccw projected
  arc A28 (8.1615, 3.8287) -> (8.4301, 3.5006) centre (13.5164, 7.9382) ccw projected
  arc A29 (8.4301, 3.5006) -> (9.5184, 3.9813) centre (7.1229, 7.9317) ccw projected
  arc A30 (9.5184, 3.9813) -> (9.7748, 3.7381) centre (13.5164, 7.9382) ccw projected
  arc A31 (9.7748, 3.7381) -> (9.3518, 2.6261) centre (13.8454, 1.5533) ccw projected
  arc A32 (9.3518, 2.6261) -> (9.6935, 2.3751) centre (13.5164, 7.9382) ccw projected
  arc A33 (9.6935, 2.3751) -> (10.6281, 3.1114) centre (7.3254, 6.3419) ccw projected
  arc A34 (10.6281, 3.1114) -> (10.9368, 2.9396) centre (13.5164, 7.9382) ccw projected
  arc A35 (10.9368, 2.9396) -> (10.8037, 1.7573) centre (15.423, 1.8357) ccw projected
  arc A36 (10.8037, 1.7573) -> (11.1971, 1.5992) centre (13.5164, 7.9382) ccw projected
  arc A37 (11.1971, 1.5992) -> (11.9192, 2.5448) centre (7.9169, 4.8524) ccw projected
  arc A38 (11.9192, 2.5448) -> (12.261, 2.4551) centre (13.5164, 7.9382) ccw projected
  arc A39 (12.261, 2.4551) -> (12.426, 1.2769) centre (16.8807, 2.5016) ccw projected
  arc A40 (12.426, 1.2769) -> (12.8465, 1.2216) centre (13.5164, 7.9382) ccw projected
  arc A41 (12.8465, 1.2216) -> (13.3107, 2.317) centre (8.8602, 3.5569) ccw projected
  arc A42 (13.3107, 2.317) -> (13.664, 2.3152) centre (13.5164, 7.9382) ccw projected
  arc A43 (13.664, 2.3152) -> (14.1169, 1.215) centre (18.1271, 3.509) ccw projected
  arc A44 (14.1169, 1.215) -> (14.5379, 1.266) centre (13.5164, 7.9382) ccw projected
  arc A45 (14.5379, 1.266) -> (14.7151, 2.4424) centre (10.0961, 2.5366) ccw projected
  arc A46 (14.7151, 2.4424) -> (15.0578, 2.5286) centre (13.5164, 7.9382) ccw projected
  arc A47 (15.0578, 2.5286) -> (15.77, 1.5756) centre (19.0837, 4.7948) ccw projected
  arc A48 (15.77, 1.5756) -> (16.1651, 1.7296) centre (13.5164, 7.9382) ccw projected
  arc A49 (16.1651, 1.7296) -> (16.0442, 2.9132) centre (11.5469, 1.8557) ccw projected
  arc A50 (16.0442, 2.9132) -> (16.3547, 3.0819) centre (13.5164, 7.9382) ccw projected
  arc A51 (16.3547, 3.0819) -> (17.2816, 2.3359) centre (19.6905, 6.2781) ccw projected
  arc A52 (17.2816, 2.3359) -> (17.6259, 2.5834) centre (13.5164, 7.9382) ccw projected
  arc A53 (17.6259, 2.5834) -> (17.2144, 3.6997) centre (13.1214, 1.557) ccw projected
  arc A54 (17.2144, 3.6997) -> (17.4733, 3.9403) centre (13.5164, 7.9382) ccw projected
  arc A55 (17.4733, 3.9403) -> (18.5565, 3.4483) centre (19.9094, 7.8657) ccw projected
  arc A56 (18.5565, 3.4483) -> (18.8285, 3.7736) centre (13.5164, 7.9382) ccw projected
  arc A57 (18.8285, 3.7736) -> (18.1523, 4.7526) centre (14.7208, 1.6593) ccw projected
  arc A58 (18.1523, 4.7526) -> (18.3432, 5.0499) centre (13.5164, 7.9382) ccw projected
  arc A59 (18.3432, 5.0499) -> (19.5148, 4.8428) centre (19.7266, 9.4579) ccw projected
  arc A60 (19.5148, 4.8428) -> (19.6973, 5.2256) centre (13.5164, 7.9382) ccw projected
  arc A61 (19.6973, 5.2256) -> (18.7989, 6.0056) centre (16.2445, 2.1561) ccw projected
  arc A62 (18.7989, 6.0056) -> (18.9098, 6.3411) centre (13.5164, 7.9382) ccw projected
  arc A63 (18.9098, 6.3411) -> (20.0961, 6.4318) centre (19.1536, 10.9546) ccw projected
  arc A64 (20.0961, 6.4318) -> (20.1777, 6.8479) centre (13.5164, 7.9382) ccw projected
  arc A65 (20.1777, 6.8479) -> (19.1136, 7.38) centre (17.5967, 3.0162) ccw projected
  arc A66 (19.1136, 7.38) -> (19.1376, 7.7325) centre (13.5164, 7.9382) ccw projected
  arc A67 (19.1376, 7.7325) -> (20.264, 8.1154) centre (18.2263, 12.2617) ccw projected
  arc A68 (20.264, 8.1154) -> (20.2396, 8.5388) centre (13.5164, 7.9382) ccw projected
  arc A69 (20.2396, 8.5388) -> (19.0766, 8.7895) centre (18.6926, 4.1855) ccw projected
  arc A70 (19.0766, 8.7895) -> (19.0122, 9.1369) centre (13.5164, 7.9382) ccw projected
  arc A71 (19.0122, 9.1369) -> (20.008, 9.788) centre (17.0032, 13.2972) ccw projected
  arc A72 (20.008, 9.788) -> (19.879, 10.1919) centre (13.5164, 7.9382) ccw projected
  arc A73 (19.879, 10.1919) -> (18.6902, 10.1455) centre (19.4633, 5.5907) ccw projected
  arc A74 (18.6902, 10.1455) -> (18.5414, 10.466) centre (13.5164, 7.9382) ccw projected
  arc A75 (18.5414, 10.466) -> (19.344, 11.3442) centre (15.5609, 13.996) ccw projected
  arc A76 (19.344, 11.3442) -> (19.1187, 11.7034) centre (13.5164, 7.9382) ccw projected
  arc A77 (19.1187, 11.7034) -> (17.9787, 11.3629) centre (19.8602, 7.1434) ccw projected
  arc A78 (17.9787, 11.3629) -> (17.7549, 11.6363) centre (13.5164, 7.9382) ccw projected
  arc A79 (17.7549, 11.6363) -> (18.3139, 12.6865) centre (13.9902, 14.3141) ccw projected
  arc A80 (18.3139, 12.6865) -> (18.0063, 12.9784) centre (13.5164, 7.9382) ccw projected
  arc A81 (18.0063, 12.9784) -> (16.9869, 12.365) centre (19.8586, 8.746) ccw projected
  arc A82 (16.9869, 12.365) -> (16.7021, 12.5742) centre (13.5164, 7.9382) ccw projected
  arc A83 (16.7021, 12.5742) -> (16.9823, 13.7304) centre (12.3897, 14.2316) ccw projected
  arc A84 (16.9823, 13.7304) -> (16.6118, 13.9366) centre (13.5164, 7.9382) ccw projected
  arc A85 (16.6118, 13.9366) -> (15.7769, 13.089) centre (19.4584, 10.2979) ccw projected
  arc A86 (15.7769, 13.089) -> (15.4491, 13.2208) centre (13.5164, 7.9382) ccw projected
  arc A87 (15.4491, 13.2208) -> (15.433, 14.4104) centre (10.86, 13.7537) ccw projected
  arc A88 (15.433, 14.4104) -> (15.0228, 14.518) centre (13.5164, 7.9382) ccw projected
  arc A89 (15.0228, 14.518) -> (14.425, 13.4894) centre (18.6849, 11.7015) ccw projected
  arc A90 (14.425, 13.4894) -> (14.0746, 13.5355) centre (13.5164, 7.9382) ccw projected
  arc A91 (14.0746, 13.5355) -> (13.7632, 14.6837) centre (9.4972, 12.9104) ccw projected
  arc A92 (13.7632, 14.6837) -> (13.3392, 14.6859) centre (13.5164, 7.9382) ccw projected
  arc A93 (13.3392, 14.6859) -> (13.0159, 13.5409) centre (17.5867, 12.8686) ccw projected
  arc A94 (13.0159, 13.5409) -> (12.6651, 13.4985) centre (13.5164, 7.9382) ccw projected
  arc A95 (12.6651, 13.4985) -> (12.0779, 14.5332) centre (8.3869, 11.7546) ccw projected
  arc A96 (12.0779, 14.5332) -> (11.6667, 14.4299) centre (13.5164, 7.9382) ccw projected
  arc A97 (11.6667, 14.4299) -> (11.6383, 13.2405) centre (16.2327, 13.726) ccw projected
  arc A98 (11.6383, 13.2405) -> (11.3091, 13.1121) centre (13.5164, 7.9382) ccw projected
  arc A99 (11.3091, 13.1121) -> (10.483, 13.9683) centre (7.599, 10.3591) ccw projected
  arc A100 (10.483, 13.9683) -> (10.1104, 13.7659) centre (13.5164, 7.9382) ccw projected
  circle A101 centre (13.5164, 7.9382) radius 6.75
  circle A102 centre (13.5164, 7.9382) radius 7.15
  line L0 (-10.0014, 27.7) -> (43.7986, 27.7) projected
  line L1 (-10.0014, 27.7) -> (-10.0014, 0) projected
  line L2 (-10.0014, 0) -> (0, 0) projected
  arc A103 (0, 0) -> (10.1832, 0) centre (5.0916, 5.5748) ccw projected
  line L3 (10.1832, 0) -> (23.789, 0) projected
  arc A104 (20.8845, 2.8543) -> (23.789, 1) centre (29.9486, 13.85) ccw projected
  arc A105 (4.3064, 18.8425) -> (1.0471, 19.1146) centre (2.9986, 22.8337) ccw projected
  arc A106 (7.5647, 12.9022) -> (4.3064, 18.8425) centre (2.2486, 13.85) ccw projected
  arc A107 (-0.906, 9.4672) -> (10.4371, 0.8262) centre (5.0916, 5.5748) ccw projected
  arc A108 (1.0471, 19.1146) -> (-0.906, 9.4672) centre (2.2486, 13.85) ccw projected
  line L4 (23.789, 0) -> (23.789, 1) projected
  arc A109 (7.5647, 12.9022) -> (10.4371, 0.8262) centre (13.5164, 7.9382) ccw projected
  line L5 (20.8845, 5.5354) -> (20.8845, 2.8543) projected
  arc A110 (20.8845, 5.5354) -> (24.0356, 3.0645) centre (29.9486, 13.85) ccw projected
  line L6 (27.7194, 7.5317) -> (24.0356, 3.0645) projected
  arc A111 (24.1705, 10.4583) -> (27.7194, 7.5317) centre (29.9486, 13.85) ccw projected
  line L7 (24.5486, 13.85) -> (24.1705, 10.4583) projected
  arc A112 (31.5107, 19.0191) -> (24.5486, 13.85) centre (29.9486, 13.85) ccw projected
  line L8 (32.1777, 20.1683) -> (31.5107, 19.0191) projected
  line L9 (35.8615, 24.6355) -> (32.1777, 20.1683) projected
  arc A113 (39.4105, 21.7089) -> (35.8615, 24.6355) centre (29.9486, 13.85) ccw projected
  line L10 (39.4105, 0) -> (39.4105, 21.7089) projected
  line L11 (43.7986, 0) -> (39.4105, 0) projected
  line L12 (43.7986, 27.7) -> (43.7986, 0) projected
  point P0 (4.2986, 27.7)
  point P1 (-7.4509, 21.8046)
  point P2 (7.7764, 12.2015)
  point P3 (10.8315, 1.3115)
  dimension "d55" = 0.4
  constraints: 1 centre point, 1 coincident, 4 other
extrude "Extrusion6" add sketch "Sketch6" along normal blind 2.6 contours A0 | A100 A99 A98 A97 A96 A95 A94 A93 A92 A91 A90 A89 A88 A87 A86 A85 A84 A83 A82 A81 A80 A79 A78 A77 A76 A75 A74 A73 A72 A71 A70 A69 A68 A67 A66 A65 A64 A63 A62 A61 A60 A59 A58 A57 A56 A55 A54 A53 A52 A51 A50 A49 A48 A47 A46 A45 A44 A43 A42 A41 A40 A39 A38 A37 A36 A35 A34 A33 A32 A31 A30 A29 A28 A27 A26 A25 A24 A23 A22 A21 A20 A19 A18 A17 A16 A15 A14 A13 A12 A11 A10 A9 A8 A7 A6 A5 A4 A3 A2 A1 | A1 A2 A3 A101 | A101 A97 A98 A99 | A5 A6 A7 A101 | A101 A93 A94 A95 | A9 A10 A11 A101 | A101 A89 A90 A91 | A13 A14 A15 A101 | A101 A85 A86 A87 | A17 A18 A19 A101 | A101 A81 A82 A83 | A21 A22 A23 A101 | A101 A77 A78 A79 | A25 A26 A27 A101 | A101 A73 A74 A75 | A29 A30 A31 A101 | A101 A69 A70 A71 | A33 A34 A35 A101 | A101 A65 A66 A67 | A37 A38 A39 A101 | A101 A61 A62 A63 | A41 A42 A43 A101 | A101 A57 A58 A59 | A45 A46 A47 A101 | A101 A53 A54 A55 | A49 A50 A51 A101 | A102 | L0 L12 L11 L10 A113 L9 L8 A112 L7 A111 L6 A110 L5 A104 L4 L3 A103 L2 L1 | A106 A109 A107 A108 A105
sketch "Sketch7" plane through (-4.2986, 24.5, 27.7) normal (0, 1, 0) x (1, 0, 0)
  circle A0 centre (28.4986, 22.8337) radius 4 projected
  circle A1 centre (28.4986, 22.8337) radius 12.5 projected
  circle A2 centre (28.4986, 22.8337) radius 4.2
  line L0 (31.5107, 19.0191) -> (32.1777, 20.1683)
  arc A3 (31.5107, 19.0191) -> (24.5486, 13.85) centre (29.9486, 13.85) ccw
  line L1 (32.1777, 20.1683) -> (31.7444, 20.1683)
  point P0 (4.2986, 27.7)
  point P1 (30.6189, 19.2082)
  dimension "d58" = 0.2
  constraints: 4 end point, 2 point on circle, 1 centre point, 1 horizontal, 3 other
extrude "Extrusion7" cut sketch "Sketch7" against normal blind 2.6 contours A0 A3 | A0 A3 A2 | A3 A0 | A0 A3 A2 | A2 L1 L0 A3